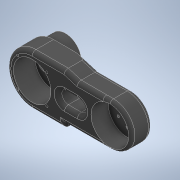
# Autodesk Inventor part: E_02
Saved by Autodesk Inventor 2021 (Build 250183000, 183)
## iProperties
Created: 2022-03-16
Part Number: E_02
Material: PETG
Document SubType Name: Modeling
Designer: Alcatraz
Density: 1.27 g/cm^3
Appearance: Genérico
Mass: 209.768 g
Surface Area: 445.039 cm^2
Volume: 165.172 cm^3
Author: Alcatraz
Autodesk Inventor part; units mm, degrees
ref_plane "YZ Plane" through (0, 0, 0) normal (1, 0, 0) x (0, 1, 0)
ref_plane "XZ Plane" through (0, 0, 0) normal (0, 1, 0) x (-1, 0, 0)
ref_plane "XY Plane" through (0, 0, 0) normal (0, 0, 1) x (1, 0, 0)
sketch "Boceto1" plane through (0, 0, 0) normal (0, 0, 1) x (1, 0, 0)
  circle A0 centre (0, 0) radius 29
  arc A1 (0, -33) -> (0, 33) centre (0, 0) ccw
  circle A2 centre (-120, 0) radius 29
  arc A3 (-120, 39) -> (-120, -39) centre (-120, 0) ccw
  line L0 (-120, 39) -> (-70, 39)
  line L1 (-120, -39) -> (-70, -39)
  line L2 (0, 33) -> (-50, 33)
  line L3 (0, -33) -> (-70, -33)
  line L4 (-70, 39) -> (-50, 33)
  line L5 (-70, -39) -> (-70, -33)
  arc A4 (-70, 10) -> (-70, -10) centre (-70, 0) ccw
  arc A5 (-50, -10) -> (-50, 10) centre (-50, 0) ccw
  line L6 (-70, 10) -> (-50, 10)
  line L7 (-70, -10) -> (-50, -10)
  dimension "DiametroEje" = 58
  dimension "d1" = 66
  dimension "DiametroCajaMotor" = 58
  dimension "d30" = 78
  dimension "LongitudEslabon" = 120
  dimension "d136" = 50
  dimension "d137" = 50
  dimension "d187" = 20
  dimension "d188" = 50
  dimension "d189" = 50
  dimension "d192" = 10
  dimension "d193" = 10
  dimension "d194" = 33
  dimension "d195" = 20
  constraints: 16 end point, 8 point on circle, 6 centre point, 6 tangent, 5 horizontal, 3 coincident, 1 horizontal alignment, 1 parallel
  measures "DiametroEje" diameter of A0
  measures "d1" diameter of A1
  measures "DiametroCajaMotor" diameter of A2
  measures "d30" diameter of A3
  measures "LongitudEslabon" distance of A0.centre A2.centre
  measures "d136" distance of L0.start L0.end
  measures "d137" distance of L2.start L2.end
  measures "d187" diameter of A5
  measures "d188" distance of A2.centre A4.centre
  measures "d189" distance of A0.centre A5.centre
  measures "d192" radius of A5
  measures "d193" radius of A4
  measures "d194" distance from line of L2 A5.centre
  measures "d195" distance of L6.start L6.end
extrude "Extrusión4" add sketch "Boceto1" along normal blind 33
extrude "Extrusión5" add sketch "Boceto1" along normal blind 6 contours A0
sketch "Boceto3" plane through (0, 0, 6) normal (0, 0, 1) x (1, 0, 0)
  circle A0 centre (0, 0) radius 20
  line L0 (0, 0) -> (0, 16)
  circle A1 centre (0, 16) radius 1.5
  dimension "d72" = 40
  dimension "d73" = 16
  dimension "d74" = 3
  constraints: 2 centre point, 2 coincident, 2 end point, 1 vertical
  measures "d72" diameter of A0
  measures "d73" distance of L0.start L0.end
  measures "d74" diameter of A1
hole "Agujero2" at (0, 16, 6) direction (0, 0, -1) diameter 3.6881 depth 13 thread size "M4.5x0.75" class "6H" standard "ISO Metric profile"
pattern_circular "Patrón circular2" count 6 over 360 about axis through (0, 0, 0) along (0, 0, 1) of "Agujero2"
sketch "Boceto4" plane through (-120, 0, 6) normal (0, 0, 1) x (1, 0, 0)
  line L0 (25, -16) -> (-25, -16)
  line L1 (-25, -16) -> (-25, 16)
  line L2 (-25, 16) -> (25, 16)
  line L3 (25, 16) -> (25, -16)
  line L4 (25, -16) -> (-25, 16) construction
  line L5 (-25, -16) -> (25, 16) construction
  circle A0 centre (-13.5, 0) radius 6
  line L6 (-1.85, 0) -> (-1.85, 10.5)
  line L7 (-1.85, 10.5) -> (5.15, 10.5)
  line L8 (5.15, 10.5) -> (5.15, -10.5)
  line L9 (5.15, -10.5) -> (-1.85, -10.5)
  line L10 (-1.85, -10.5) -> (-1.85, 0)
  line L11 (15.266, 4) -> (12.466, 4)
  line L12 (11.666, 4.8) -> (11.666, 9.2)
  line L13 (12.466, 10) -> (18.066, 10)
  line L14 (18.866, 9.2) -> (18.866, 4.8)
  line L15 (18.066, 4) -> (15.266, 4)
  line L16 (15.266, -4) -> (12.466, -4)
  line L17 (11.666, -4.8) -> (11.666, -9.2)
  line L18 (12.466, -10) -> (18.066, -10)
  line L19 (18.866, -9.2) -> (18.866, -4.8)
  line L20 (18.066, -4) -> (12.466, -4)
  arc A1 (11.666, -9.2) -> (12.466, -10) centre (12.466, -9.2) ccw
  arc A2 (12.466, -4) -> (11.666, -4.8) centre (12.466, -4.8) ccw
  arc A3 (18.866, -4.8) -> (18.066, -4) centre (18.066, -4.8) ccw
  arc A4 (18.066, -10) -> (18.866, -9.2) centre (18.066, -9.2) ccw
  arc A5 (18.066, 4) -> (18.866, 4.8) centre (18.066, 4.8) ccw
  arc A6 (18.866, 9.2) -> (18.066, 10) centre (18.066, 9.2) ccw
  arc A7 (12.466, 10) -> (11.666, 9.2) centre (12.466, 9.2) ccw
  arc A8 (11.666, 4.8) -> (12.466, 4) centre (12.466, 4.8) ccw
  circle A9 centre (22.5, -8) radius 1
  circle A10 centre (22.5, 8) radius 1
  circle A11 centre (17, -13.5) radius 1
  circle A12 centre (-7, -13.5) radius 1
  circle A13 centre (1, -13.5) radius 1
  circle A14 centre (9, -13.5) radius 1
  circle A15 centre (17, 13.5) radius 1
  circle A16 centre (-7, 13.5) radius 1
  circle A17 centre (1, 13.5) radius 1
  circle A18 centre (9, 13.5) radius 1
  point P0 (120, 0)
  dimension "d85" = 50
  dimension "d86" = 32
  dimension "d87" = 12
  dimension "d88" = 11.65
  dimension "d89" = 10.5
  dimension "d90" = 7
  dimension "d91" = 21
  dimension "d92" = 2.8
  dimension "d93" = 4.4
  dimension "d94" = 5.6
  dimension "d95" = 4.4
  dimension "d96" = 0.8
  dimension "d97" = 0.8
  dimension "d98" = 0.8
  dimension "d99" = 0.8
  dimension "d100" = 0.8
  dimension "d101" = 0.8
  dimension "d102" = 2
  dimension "d103" = 2
  dimension "d104" = 2
  dimension "d105" = 2
  dimension "d106" = 2
  dimension "d107" = 2
  dimension "d108" = 2
  dimension "d109" = 2
  dimension "d110" = 2
  dimension "d111" = 2
  constraints: 42 end point, 19 centre point, 16 point on circle, 5 perpendicular, 4 tangent, 2 parallel, 2 point on line, 1 collinear
  measures "d85" distance of L2.start L3.start
  measures "d86" distance of L0.end L2.start
  measures "d87" diameter of A0
  measures "d88" distance of A0.centre L10.end
  measures "d89" distance of L10.end L6.end
  measures "d90" distance of L6.end L8.start
  measures "d91" distance of L8.start L9.start
  measures "d92" distance of L11.start L11.end
  measures "d93" distance of L12.start L12.end
  measures "d94" distance of L13.start L13.end
  measures "d95" distance of L17.start L17.end
  measures "d96" radius of A2
  measures "d97" radius of A3
  measures "d98" radius of A4
  measures "d99" radius of A5
  measures "d100" radius of A6
  measures "d101" radius of A8
  measures "d102" diameter of A9
  measures "d103" diameter of A10
  measures "d104" diameter of A11
  measures "d105" diameter of A12
  measures "d106" diameter of A13
  measures "d107" diameter of A14
  measures "d108" diameter of A15
  measures "d109" diameter of A16
  measures "d110" diameter of A17
  measures "d111" diameter of A18
fillet "Empalme5" radius 6 13 edges at (33, 0, 33) (-35, -33, 33) (-25, 33, 33) (33, 0, 0) (-35, -33, 0) (-25, 33, 0) (-60, 36, 0) (-70, -36, 0) (-70, -36, 33) (-60, 36, 33) (-95, -39, 33) (-95, 39, 33) (-159, 0, 33)
fillet "Empalme6" radius 6 4 edges at (-40, 0, 33) (-80, 0, 33) (-40, 0, 0) (-80, 0, 0)
sketch "Boceto6" plane through (0, 0, 0) normal (0, 0, -1) x (-1, 0, 0)
  circle A0 centre (120, 0) radius 29 projected
  circle A1 centre (120, 0) radius 35
  line L0 (120, 0) -> (142.6274, -22.6274)
  line L1 (120, 0) -> (152, 0) construction
  circle A2 centre (142.6274, -22.6274) radius 1.5
  circle A3 centre (142.6274, 22.6274) radius 1.5
  circle A4 centre (97.3726, 22.6274) radius 1.5
  circle A5 centre (97.3726, -22.6274) radius 1.5
  point P0 (0, 0)
  dimension "d196" = 70
  dimension "d197" = 32
  dimension "d198" = 45
  dimension "d199" = 3
  dimension "d202" = 360
  constraints: 5 centre point, 4 end point, 2 coincident, 1 equal length, 1 horizontal, 9 other
  measures "d196" diameter of A1
  measures "d197" distance of L0.start L0.end
  measures "d198" angle of L0 L1
  measures "d199" diameter of A2
sketch "Boceto7" plane through (0, 0, 33) normal (0, 0, 1) x (1, 0, 0)
  circle A0 centre (-120, 0) radius 29 projected
  circle A1 centre (-120, 0) radius 30
  point P0 (0, 0)
  dimension "d213" = 60
  constraints: 1 centre point, 1 coincident
  measures "d213" diameter of A1
sketch "Boceto10" plane through (0, 0, 33) normal (0, 0, 1) x (1, 0, 0)
  circle A0 centre (-157.3726, -22.6274) radius 2
  circle A1 centre (-157.2184, 22.4732) radius 2
  circle A2 centre (-202.319, 22.6274) radius 2
  circle A3 centre (-202.4732, -22.4732) radius 2
  point P0 (0, 0)
  point P1 (-179.8458, 0)
  dimension "d282" = 360
  constraints: 4 centre point, 9 other
sketch "Boceto11" plane through (0, 0, 0) normal (0, 0, -1) x (-1, 0, 0)
  circle A0 centre (120, 0) radius 29 projected
  circle A1 centre (120, 0) radius 30
  circle A2 centre (120, 0) radius 29
  line L0 (120, 0) -> (0, 0)
  point P0 (198.1904, 22.5856)
  point P1 (198.1904, -22.5856)
  dimension "d284" = 60
  dimension "d387" = 120
  constraints: 2 centre point, 2 coincident, 2 end point, 1 horizontal, 1 other
  measures "d284" diameter of A1
  measures "d387" distance of L0.start L0.end
extrude "Extrusión15" add sketch "Boceto11" along normal blind 3 contours A0 | A1
sketch "Boceto12" plane through (-120, 0, 0) normal (0, 0, 1) x (1, 0, 0)
  circle A0 centre (-7, 13.5) radius 1.1
  circle A1 centre (1, 13.5) radius 1.1
  line L0 (15.65, 11.657) -> (-6.356, 11.657)
  line L1 (15.65, -11.657) -> (-6.356, -11.657)
  line L2 (25, 16) -> (-25, -16) construction
  line L3 (25, -16) -> (-25, 16) construction
  line L4 (-25, -16) -> (25, -16)
  line L5 (-25, 16) -> (-25, -16)
  line L6 (25, -16) -> (25, 16)
  circle A2 centre (9, 13.5) radius 1.1
  line L7 (25, 16) -> (-25, 16)
  line L8 (25, 0) -> (19, 0)
  line L9 (19, 0) -> (19, 8.307)
  arc A3 (19, 8.307) -> (18.2, 9.107) centre (18.2, 8.307) ccw
  circle A4 centre (22.5, 8) radius 1.1
  arc A5 (16.45, 10.857) -> (18.2, 9.107) centre (18.2, 10.857) ccw
  arc A6 (16.45, 10.857) -> (15.65, 11.657) centre (15.65, 10.857) ccw
  circle A7 centre (17, 13.5) radius 1.1
  arc A8 (-6.356, -9.015) -> (-6.356, 9.015) centre (-13.002, 0) ccw
  arc A9 (-7.156, -10.857) -> (-6.356, -11.657) centre (-6.356, -10.857) ccw
  circle A10 centre (-7, -13.5) radius 1.1
  circle A11 centre (1, -13.5) radius 1.1
  arc A12 (-6.356, 11.657) -> (-7.156, 10.857) centre (-6.356, 10.857) ccw
  line L10 (-7.156, -10.857) -> (-7.156, -9.815)
  line L11 (-7.156, 10.857) -> (-7.156, 9.815)
  arc A13 (-6.356, -9.015) -> (-7.156, -9.815) centre (-6.356, -9.815) ccw
  arc A14 (-7.156, 9.815) -> (-6.356, 9.015) centre (-6.356, 9.815) ccw
  circle A15 centre (-13.5, 0) radius 11.5
  line L12 (19, 0) -> (19, -8.307)
  circle A16 centre (22.5, -8) radius 1.1
  arc A17 (18.2, -9.107) -> (16.45, -10.857) centre (18.2, -10.857) ccw
  arc A18 (15.65, -11.657) -> (16.45, -10.857) centre (15.65, -10.857) ccw
  circle A19 centre (9, -13.5) radius 1.1
  circle A20 centre (17, -13.5) radius 1.1
  arc A21 (18.2, -9.107) -> (19, -8.307) centre (18.2, -8.307) ccw
  point P0 (120, 0)
  point P1 (0, 0)
  point P2 (-6.36, 9.015)
  point P3 (-7.116, 9.5653)
  point P4 (-7.116, -9.5653)
  point P5 (-6.36, -9.015)
  dimension "d287" = 32
  dimension "d288" = 50
  dimension "d289" = 23
  dimension "d290" = 11.5
  dimension "d291" = 2.2
  dimension "d292" = 2.2
  dimension "d293" = 2.2
  dimension "d294" = 2.2
  dimension "d295" = 2.2
  dimension "d296" = 2.2
  dimension "d297" = 2.2
  dimension "d298" = 2.2
  dimension "d299" = 2.2
  dimension "d300" = 2.2
  dimension "d301" = 27
  dimension "d302" = 16
  dimension "d303" = 8
  dimension "d304" = 13.5
  dimension "d305" = 13.5
  dimension "d306" = 8
  dimension "d307" = 8
  dimension "d308" = 8
  dimension "d309" = 8
  dimension "d310" = 8
  dimension "d311" = 8
  dimension "d312" = 6
  dimension "d313" = 8.307
  dimension "d314" = 22.006
  dimension "d315" = 1.042
  dimension "d316" = 1.042
  dimension "d317" = 11.2
  dimension "d318" = 0.8
  dimension "d319" = 0.8
  dimension "d320" = 0.8
  dimension "d321" = 0.8
  dimension "d322" = 1.75
  dimension "d323" = 0.8
  dimension "d324" = 1.75
  dimension "d325" = 0.8
  constraints: 26 end point, 23 point on circle, 22 centre point, 3 midpoint, 3 tangent, 2 parallel, 1 perpendicular
  measures "d287" distance of L5.end L7.end
  measures "d288" distance of L7.end L7.start
  measures "d289" diameter of A15
  measures "d290" distance from line of L5 A15.centre
  measures "d291" diameter of A16
  measures "d292" diameter of A4
  measures "d293" diameter of A7
  measures "d294" diameter of A20
  measures "d295" diameter of A19
  measures "d296" diameter of A11
  measures "d297" diameter of A10
  measures "d298" diameter of A0
  measures "d299" diameter of A1
  measures "d300" diameter of A2
  measures "d301" distance of A7.centre A20.centre
  measures "d302" distance of A4.centre A16.centre
  measures "d303" vertical distance of A16.centre A15.centre
  measures "d304" vertical distance of A20.centre A15.centre
  measures "d305" vertical distance of A10.centre A15.centre
  measures "d306" distance of A1.centre A0.centre
  measures "d307" distance of A2.centre A1.centre
  measures "d308" distance of A7.centre A2.centre
  measures "d309" distance of A19.centre A20.centre
  measures "d310" distance of A19.centre A11.centre
  measures "d311" distance of A10.centre A11.centre
  measures "d312" distance of L8.start L12.start
  measures "d313" distance of L12.start L12.end
  measures "d314" distance of L1.start L1.end
  measures "d315" distance of L11.start L11.end
  measures "d316" distance of L10.start L10.end
  measures "d317" radius of A8
  measures "d318" radius of A14
  measures "d319" radius of A12
  measures "d320" radius of A13
  measures "d321" radius of A6
  measures "d322" radius of A5
  measures "d323" radius of A3
  measures "d324" radius of A17
  measures "d325" radius of A18
extrude "Extrusión16" cut sketch "Boceto12" against normal blind 3 contours A14 A15 A13 | A8 A15
extrude "Extrusión17" cut sketch "Boceto12" against normal blind 2.4 contours A6 A5 A3 L9 L12 A21 A17 A18 L1 A9 L10 A13 A15 A8 A14 L11 A12 L0
sketch "Boceto14" plane through (-120, 0, -3) normal (0, 0, -1) x (-1, 0, 0)
  arc A0 (7.116, -9.5653) -> (7.116, 9.5653) centre (13.5, 0) ccw projected
  circle A1 centre (13.5, 0) radius 20.6175
  circle A2 centre (13.5, 0) radius 24.6175
  circle A3 centre (0, 0) radius 30 projected
  arc A4 (17.6381, -24.2672) -> (17.6381, 24.2672) centre (0, 0) ccw
  point P0 (-120, 0)
  dimension "DiametroRodamiento" = 41.235
  dimension "d367" = 49.235
  constraints: 6 point on circle, 3 centre point, 2 coincident
  measures "DiametroRodamiento" diameter of A1
  measures "d367" diameter of A2
extrude "Extrusión19" add sketch "Boceto14" against normal blind 3 contours A1 A3 | A1 A3 A2 picked at (31.015, -3.4548) picked at (36.4195, 3.2884)
extrude "Extrusión20" add sketch "Boceto14" along normal blind 28.934 contours A1 A3 A2 | A1 A3 A2
sketch "Boceto15" plane through (0, 0, 33) normal (0, 0, 1) x (1, 0, 0)
  circle A0 centre (-120, 0) radius 29 projected
  circle A1 centre (-120, 0) radius 29
  line L0 (-120, 0) -> (-142.6274, -22.6274)
  line L1 (-120, 0) -> (-88, 0) construction
  circle A2 centre (-142.6274, -22.6274) radius 1.5
  circle A3 centre (-97.3726, -22.6274) radius 1.5
  circle A4 centre (-97.3726, 22.6274) radius 1.5
  circle A5 centre (-142.6274, 22.6274) radius 1.5
  point P0 (0, 0)
  dimension "d372" = 58
  dimension "d373" = 32
  dimension "d374" = 135
  dimension "d375" = 3
  dimension "d378" = 360
  constraints: 5 centre point, 4 end point, 2 coincident, 1 equal length, 1 horizontal, 9 other
  measures "d372" diameter of A1
  measures "d373" distance of L0.start L0.end
  measures "d374" angle of L0 L1
  measures "d375" diameter of A2
hole "Agujero7" at (-97.3726, -22.6274, 33) at (-97.3726, 22.6274, 33) at (-142.6274, -22.6274, 33) at (-142.6274, 22.6274, 33) direction (0, 0, -1) diameter 3.6881 depth 13 thread size "M4.5x0.75" class "6H" standard "ISO Metric profile"
sketch "Boceto16" plane through (0, 0, 6) normal (0, 0, 1) x (1, 0, 0)
  circle A0 centre (0, 0) radius 6.868
  dimension "d388" = 13.736
  constraints: 1 centre point, 1 coincident
  measures "d388" diameter of A0
extrude "Extrusión21" cut sketch "Boceto16" against normal blind 22.934
hole "Agujero8" at (-111, -13.5, 0) at (-111, 13.5, 0) at (-103, -13.5, 0) at (-97.5, -8, 0) at (-97.5, 8, 0) at (-103, 13.5, 0) direction (0, 0, -1) diameter 2.1129 depth 7.8 tip angle 118 thread size "M2.6x0.45" class "6H" standard "ANSI Metric M Profile"
sketch "Boceto17" plane through (-133.5, 0, -3) normal (0, 0, -1) x (-1, 0, 0)
  arc A0 (-6.384, -9.5653) -> (-6.384, 9.5653) centre (0, 0) ccw projected
  circle A1 centre (0, 0) radius 11.5
  circle A2 centre (0, 0) radius 20.6175
  point P0 (-133.5, 0)
  point P1 (-6.384, -9.5653)
  point P2 (-6.384, 9.5653)
  constraints: 2 centre point, 2 coincident
extrude "Extrusión22" add sketch "Boceto17" along normal blind 6
sketch "Boceto18" plane through (0, 0, 0) normal (0, 0, -1) x (-1, 0, 0)
  arc A0 (137.6381, 24.2672) -> (137.6381, -24.2672) centre (120, 0) ccw projected
  arc A1 (142.2307, 23.0173) -> (142.2307, -23.0173) centre (120, 0) ccw
  arc A2 (137.6381, -24.2672) -> (137.6381, 24.2672) centre (133.5, 0) ccw projected
  arc A3 (142.2307, 23.0173) -> (137.6381, 24.2672) centre (133.5, 0) ccw
  arc A4 (137.6381, -24.2672) -> (142.2307, -23.0173) centre (133.5, 0) ccw
  point P0 (0, 0)
  dimension "d400" = 64
  constraints: 8 point on circle, 3 centre point, 1 coincident
  measures "d400" diameter of A1
extrude "Extrusión23" add sketch "Boceto18" along normal blind 3 contours A0 A2 A1
fillet "Empalme7" radius 2 2 edges at (-88, 0, 0) (-158.1175, 0, 0)
